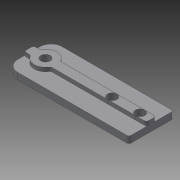
# Autodesk Inventor part: adapter_50mm
Saved by Autodesk Inventor 2013 (Build 170138000, 138)
## iProperties
Created: 2014-01-29
Part Number: adapter_50mm
Material: Ogólny
Document SubType Name: Modeling
Designer: Piotr
Density: 1 g/cm^3
Author: Piotr
Autodesk Inventor part; units mm, degrees
ref_plane "YZ Plane" through (0, 0, 0) normal (1, 0, 0) x (0, 1, 0)
ref_plane "XZ Plane" through (0, 0, 0) normal (0, 1, 0) x (-1, 0, 0)
ref_plane "XY Plane" through (0, 0, 0) normal (0, 0, 1) x (1, 0, 0)
sketch "Szkic1" plane through (0, 0, 0) normal (0, 0, 1) x (1, 0, 0)
  line L0 (55, -20) -> (-55, -20)
  line L1 (-55, -20) -> (-55, 20)
  line L2 (-55, 20) -> (55, 20)
  line L3 (55, 20) -> (55, -20)
  line L4 (55, -20) -> (-55, 20) construction
  line L5 (-55, -20) -> (55, 20) construction
  line L6 (-55, 0) -> (55, 0) construction
  line L7 (-55, -4.25) -> (55, -4.25)
  line L8 (55, -4.25) -> (55, 4.25)
  line L9 (55, 4.25) -> (-55, 4.25)
  line L10 (-55, 4.25) -> (-55, -4.25)
  line L11 (-55, -4.25) -> (55, 4.25) construction
  line L12 (55, -4.25) -> (-55, 4.25) construction
  circle A0 centre (-40, 0) radius 10
  point P0 (0, 0)
  point P1 (0, 0)
  point P2 (-40, 0)
  point P3 (20, 0)
  point P4 (45, 0)
  dimension "d1" = 40
  dimension "d4" = 8.5
  dimension "d9" = 15
  dimension "d12" = 10
  dimension "d31" = 95
  dimension "d32" = 25
  dimension "d33" = 20
  constraints: 26 end point, 7 midpoint, 4 parallel, 3 point on line, 2 collinear, 2 horizontal, 2 perpendicular, 1 centre point, 1 coincident
  measures "d1" distance of L0.end L1.end
  measures "d4" distance of L8.end L7.end
  measures "d9" distance from line of L1 point (-40, 0)
  measures "d12" distance from line of L3 point (45, 0)
  measures "d31" distance from line of L3 point (-40, 0)
  measures "d32" distance of point (20, 0) point (45, 0)
  measures "d33" diameter of A0
extrude "Wyciągnięcie proste1" add sketch "Szkic1" against normal blind 6
extrude "Wyciągnięcie proste2" add sketch "Szkic1" along normal blind 3.5 contours L7 A0 L9 L3 | L1 L9 A0 L7 | A0 L7 | L7 A0 L9 | L9 A0
fillet "Zaokrąglenie1" radius 2 10 edges at (55, 4.25, 1.75) (55, -4.25, 1.75) (55, 20, -3) (55, -20, -3) (-55, -4.25, 1.75) (-55, 4.25, 1.75) (-49.0519, -4.25, 1.75) (-30.9481, -4.25, 1.75) (-30.9481, 4.25, 1.75) (-49.0519, 4.25, 1.75)
fillet "Zaokrąglenie2" radius 10 2 edges at (-55, -20, -3) (-55, 20, -3)
hole "Otwór1" at (-40, 0, 0) at (20, 0, 0) at (45, 0, 0) direction (0, 0, -1) diameter 8.5 end through all
hole "Otwór2" at (45, 0, 0) at (20, 0, 0) at (-40, 0, 0) direction (0, 0, 1) diameter 8.5 end through all
